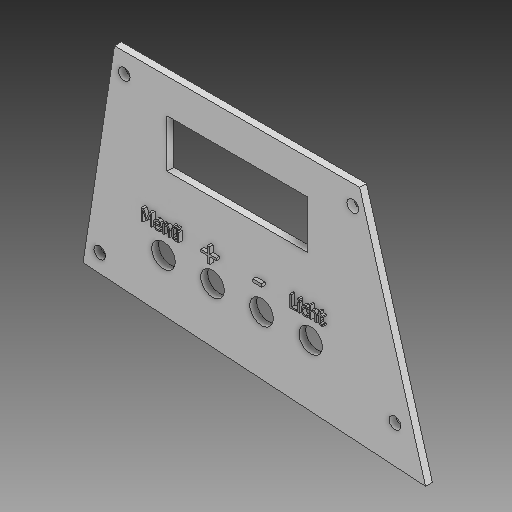
# Autodesk Inventor part: Bauteil1
Saved by Autodesk Inventor 2021 (Build 250183000, 183)
## iProperties
Created: 2021-11-26
Part Number: Bauteil1
Material: Generisch
Document SubType Name: Modeling
Designer: stroh
Density: 1 g/cm^3
Appearance: Vorgabe
Stock Number: Bedienelement
Author: stroh
Autodesk Inventor part; units mm, degrees
ref_plane "YZ Plane" through (0, 0, 0) normal (1, 0, 0) x (0, 1, 0)
ref_plane "XZ Plane" through (0, 0, 0) normal (0, 1, 0) x (-1, 0, 0)
ref_plane "XY Plane" through (0, 0, 0) normal (0, 0, 1) x (1, 0, 0)
sketch "Skizze1" plane through (0, 0, 0) normal (0, 0, 1) x (1, 0, 0)
  line L0 (-76.5913, -13.7675) -> (98.0346, -25.2043)
  line L1 (98.0346, -25.2043) -> (64.4493, 90)
  line L2 (64.4493, 90) -> (-60.5507, 90)
  line L3 (-60.5507, 90) -> (-76.5913, -13.7675)
  point P0 (0, 0)
  dimension "d0" = 175
  dimension "d1" = 120
  dimension "d2" = 105
  dimension "d3" = 125
  dimension "d5" = 70
  dimension "d12" = 90
  dimension "d14" = 90
  constraints: 8 end point
  measures "d0" distance of L0.start L0.end
  measures "d1" distance of L0.end L1.end
  measures "d2" distance of L2.end L0.start
  measures "d3" distance of L1.end L2.end
  measures "d5" angle of L1 L0
  measures "d12" vertical distance of point (0, 0) L1.end
  measures "d14" vertical distance of point (0, 0) L2.end
extrude "Extrusion1" add sketch "Skizze1" along normal blind 3.5
sketch "Skizze2" plane through (0, 0, 3.5) normal (0, 0, 1) x (1, 0, 0)
  line L0 (-33.8007, 72.5) -> (37.6993, 72.5)
  line L1 (37.6993, 72.5) -> (37.6993, 48)
  line L2 (37.6993, 48) -> (-33.8007, 48)
  line L3 (-33.8007, 48) -> (-33.8007, 72.5)
  line L4 (64.4493, 90) -> (-60.5507, 90) projected
  circle A0 centre (-35.5507, 10) radius 6.025
  circle A1 centre (-10.5507, 10) radius 6.025
  circle A2 centre (14.4493, 10) radius 6.025
  circle A3 centre (39.4493, 10) radius 6.025
  point P0 (0, 0)
  dimension "d8" = 71.5
  dimension "d9" = 24.5
  dimension "d18" = 80
  dimension "d19" = 25
  dimension "d20" = 25
  dimension "d21" = 25
  dimension "d22" = 80
  dimension "d25" = 12.05
  dimension "d26" = 12.05
  dimension "d27" = 12.05
  dimension "d28" = 12.05
  dimension "d48" = 26.75
  dimension "d49" = 26.75
  dimension "d50" = 25
  dimension "d51" = 25
  dimension "d52" = 80
  dimension "d53" = 80
  constraints: 8 end point, 4 centre point, 2 parallel, 1 horizontal, 1 perpendicular
  measures "d8" distance of L0.start L0.end
  measures "d9" distance of L2.end L0.start
  measures "d18" vertical distance of L4.end A0.centre
  measures "d19" distance of A1.centre A0.centre
  measures "d20" distance of A2.centre A1.centre
  measures "d21" distance of A2.centre A3.centre
  measures "d22" distance from line of L4 A1.centre
  measures "d25" diameter of A0
  measures "d26" diameter of A1
  measures "d27" diameter of A2
  measures "d28" diameter of A3
  measures "d48" distance from line of L4.end L3
  measures "d49" distance from line of L4.start L1
  measures "d50" horizontal distance of L4.end A0.centre
  measures "d51" horizontal distance of L4.start A3.centre
  measures "d52" distance from line of L4 A2.centre
  measures "d53" distance from line of L4 A3.centre
extrude "Extrusion2" cut sketch "Skizze2" against normal blind 5
sketch "Skizze3" plane through (0, 0, 3.5) normal (0, 0, 1) x (1, 0, 0)
  line L0 (-45.7172, 27.2505) -> (-25.2588, 27.2505) construction
  line L1 (-25.2588, 27.2505) -> (-25.2588, 20.6661) construction
  line L2 (-25.2588, 20.6661) -> (-45.7172, 20.6661) construction
  line L3 (-45.7172, 20.6661) -> (-45.7172, 27.2505) construction
  line L4 (-15.8595, 27.2834) -> (0.8474, 27.2834) construction
  line L5 (0.8474, 27.2834) -> (0.8474, 22.6055) construction
  line L6 (0.8474, 22.6055) -> (-15.8595, 22.6055) construction
  line L7 (-15.8595, 22.6055) -> (-15.8595, 27.2834) construction
  line L8 (10.9705, 24.1223) -> (26.0544, 24.1223) construction
  line L9 (26.0544, 24.1223) -> (26.0544, 18.2033) construction
  line L10 (26.0544, 18.2033) -> (10.9705, 18.2033) construction
  line L11 (10.9705, 18.2033) -> (10.9705, 24.1223) construction
  line L12 (29.9728, 27.2179) -> (48.0162, 27.2179) construction
  line L13 (48.0162, 27.2179) -> (48.0162, 20.9171) construction
  line L14 (48.0162, 20.9171) -> (29.9728, 20.9171) construction
  line L15 (29.9728, 20.9171) -> (29.9728, 27.2179) construction
  line L16 (-81.6927, 20.4062) -> (40.124, 20.4062) construction
  line L17 (-39.8693, 21.106) -> (-40.68, 21.106)
  line L18 (-40.68, 21.106) -> (-40.68, 26.3607)
  line L19 (-40.68, 26.3607) -> (-42.2718, 22.7867)
  line L20 (-42.2718, 22.7867) -> (-42.7661, 22.7867)
  line L21 (-42.7661, 22.7867) -> (-44.343, 26.3607)
  line L22 (-44.343, 26.3607) -> (-44.343, 21.106)
  line L23 (-44.343, 21.106) -> (-45.0993, 21.106)
  line L24 (-45.0993, 21.106) -> (-45.0993, 27.206)
  line L25 (-45.0993, 27.206) -> (-43.992, 27.206)
  line L26 (-43.992, 27.206) -> (-42.4695, 23.81)
  line L27 (-42.4695, 23.81) -> (-40.9964, 27.206)
  line L28 (-40.9964, 27.206) -> (-39.8693, 27.206)
  line L29 (-39.8693, 27.206) -> (-39.8693, 21.106)
  spline S0 degree 2 poles (-36.7056, 21.0022) (-37.803, 21.0022) (-39.0092, 22.2331) (-39.0092, 23.37) knots 0 0 0 1 2 2 2
  spline S1 degree 2 poles (-39.0092, 23.37) (-39.0092, 24.4872) (-37.8376, 25.812) (-36.8935, 25.812) knots 0 0 0 1 2 2 2
  spline S2 degree 2 poles (-36.8935, 25.812) (-36.4684, 25.812) (-35.8109, 25.5648) (-35.5687, 25.3028) knots 0 0 0 1 2 2 2
  spline S3 degree 2 poles (-35.5687, 25.3028) (-35.3215, 25.0408) (-35.0595, 24.2845) (-35.0595, 23.7358) knots 0 0 0 1 2 2 2
  line L30 (-35.0595, 23.7358) -> (-35.0595, 23.3156)
  line L31 (-35.0595, 23.3156) -> (-38.2282, 23.3156)
  spline S4 degree 2 poles (-38.2282, 23.3156) (-38.2282, 22.5198) (-37.4274, 21.6745) (-36.7155, 21.6745) knots 0 0 0 1 2 2 2
  spline S5 degree 2 poles (-36.7155, 21.6745) (-36.4634, 21.6745) (-35.974, 21.7882) (-35.7763, 21.8771) knots 0 0 0 1 2 2 2
  spline S6 degree 2 poles (-35.7763, 21.8771) (-35.5687, 21.976) (-35.282, 22.149) (-35.1881, 22.2281) knots 0 0 0 1 2 2 2
  line L32 (-35.1881, 22.2281) -> (-35.1436, 22.2281)
  line L33 (-35.1436, 22.2281) -> (-35.1436, 21.3878)
  spline S7 degree 2 poles (-35.1436, 21.3878) (-35.277, 21.3334) (-35.6824, 21.1752) (-35.8406, 21.1307) knots 0 0 0 1 2 2 2
  spline S8 degree 2 poles (-35.8406, 21.1307) (-36.063, 21.0664) (-36.4288, 21.0022) (-36.7056, 21.0022) knots 0 0 0 1 2 2 2
  spline S9 degree 2 poles (-35.8109, 23.9039) (-35.8208, 24.2153) (-35.9493, 24.6701) (-36.0729, 24.8233) knots 0 0 0 1 2 2 2
  spline S10 degree 2 poles (-36.0729, 24.8233) (-36.2064, 24.9963) (-36.6265, 25.1792) (-36.938, 25.1792) knots 0 0 0 1 2 2 2
  spline S11 degree 2 poles (-36.938, 25.1792) (-37.2445, 25.1792) (-37.6745, 24.9963) (-37.8525, 24.8184) knots 0 0 0 1 2 2 2
  spline S12 degree 2 poles (-37.8525, 24.8184) (-38.0255, 24.6355) (-38.2034, 24.1955) (-38.2282, 23.9039) knots 0 0 0 1 2 2 2
  line L34 (-38.2282, 23.9039) -> (-35.8109, 23.9039)
  line L35 (-30.6847, 21.106) -> (-31.4559, 21.106)
  line L36 (-31.4559, 21.106) -> (-31.4559, 23.716)
  spline S13 degree 2 poles (-31.4559, 23.716) (-31.4559, 24.0324) (-31.5152, 24.5762) (-31.6042, 24.7393) knots 0 0 0 1 2 2 2
  spline S14 degree 2 poles (-31.6042, 24.7393) (-31.6981, 24.9123) (-32.0342, 25.0804) (-32.321, 25.0804) knots 0 0 0 1 2 2 2
  spline S15 degree 2 poles (-32.321, 25.0804) (-32.6077, 25.0804) (-33.2157, 24.7739) (-33.5073, 24.5267) knots 0 0 0 1 2 2 2
  line L37 (-33.5073, 24.5267) -> (-33.5073, 21.106)
  line L38 (-33.5073, 21.106) -> (-34.2785, 21.106)
  line L39 (-34.2785, 21.106) -> (-34.2785, 25.6835)
  line L40 (-34.2785, 25.6835) -> (-33.5073, 25.6835)
  line L41 (-33.5073, 25.6835) -> (-33.5073, 25.1743)
  spline S16 degree 2 poles (-33.5073, 25.1743) (-33.1613, 25.4857) (-32.494, 25.812) (-32.1183, 25.812) knots 0 0 0 1 2 2 2
  spline S17 degree 2 poles (-32.1183, 25.812) (-31.446, 25.812) (-30.6847, 24.9222) (-30.6847, 24.0769) knots 0 0 0 1 2 2 2
  line L42 (-30.6847, 24.0769) -> (-30.6847, 21.106)
  line L43 (-26.043, 21.106) -> (-26.8141, 21.106)
  line L44 (-26.8141, 21.106) -> (-26.8141, 21.6102)
  spline S18 degree 2 poles (-26.8141, 21.6102) (-27.1701, 21.2988) (-27.8077, 20.9775) (-28.2032, 20.9775) knots 0 0 0 1 2 2 2
  spline S19 degree 2 poles (-28.2032, 20.9775) (-28.4998, 20.9775) (-29.0287, 21.1752) (-29.2215, 21.3878) knots 0 0 0 1 2 2 2
  spline S20 degree 2 poles (-29.2215, 21.3878) (-29.4193, 21.6003) (-29.6368, 22.2479) (-29.6368, 22.7125) knots 0 0 0 1 2 2 2
  line L45 (-29.6368, 22.7125) -> (-29.6368, 25.6835)
  line L46 (-29.6368, 25.6835) -> (-28.8656, 25.6835)
  line L47 (-28.8656, 25.6835) -> (-28.8656, 23.0734)
  spline S21 degree 2 poles (-28.8656, 23.0734) (-28.8656, 22.7076) (-28.8112, 22.2281) (-28.7173, 22.0501) knots 0 0 0 1 2 2 2
  spline S22 degree 2 poles (-28.7173, 22.0501) (-28.6234, 21.8722) (-28.3021, 21.7091) (-28.0005, 21.7091) knots 0 0 0 1 2 2 2
  spline S23 degree 2 poles (-28.0005, 21.7091) (-27.7188, 21.7091) (-27.0811, 22.0304) (-26.8141, 22.2627) knots 0 0 0 1 2 2 2
  line L48 (-26.8141, 22.2627) -> (-26.8141, 25.6835)
  line L49 (-26.8141, 25.6835) -> (-26.043, 25.6835)
  line L50 (-26.043, 25.6835) -> (-26.043, 21.106)
  line L51 (-26.562, 26.4497) -> (-27.3876, 26.4497)
  line L52 (-27.3876, 26.4497) -> (-27.3876, 27.2505)
  line L53 (-27.3876, 27.2505) -> (-26.562, 27.2505)
  line L54 (-26.562, 27.2505) -> (-26.562, 26.4497)
  line L55 (-28.2526, 26.4497) -> (-29.0782, 26.4497)
  line L56 (-29.0782, 26.4497) -> (-29.0782, 27.2505)
  line L57 (-29.0782, 27.2505) -> (-28.2526, 27.2505)
  line L58 (-28.2526, 27.2505) -> (-28.2526, 26.4497)
  line L59 (-6.9049, 22.8183) -> (-10.2922, 22.8183)
  line L60 (-10.2922, 22.8183) -> (-10.2922, 19.4309)
  line L61 (-10.2922, 19.4309) -> (-11.4105, 19.4309)
  line L62 (-11.4105, 19.4309) -> (-11.4105, 22.8183)
  line L63 (-11.4105, 22.8183) -> (-14.7979, 22.8183)
  line L64 (-14.7979, 22.8183) -> (-14.7979, 23.8961)
  line L65 (-14.7979, 23.8961) -> (-11.4105, 23.8961)
  line L66 (-11.4105, 23.8961) -> (-11.4105, 27.2834)
  line L67 (-11.4105, 27.2834) -> (-10.2922, 27.2834)
  line L68 (-10.2922, 27.2834) -> (-10.2922, 23.8961)
  line L69 (-10.2922, 23.8961) -> (-6.9049, 23.8961)
  line L70 (-6.9049, 23.8961) -> (-6.9049, 22.8183)
  line L71 (16.2412, 22.6636) -> (11.6999, 22.6636)
  line L72 (11.6999, 22.6636) -> (11.6999, 24.1223)
  line L73 (11.6999, 24.1223) -> (16.2412, 24.1223)
  line L74 (16.2412, 24.1223) -> (16.2412, 22.6636)
  line L75 (34.1252, 20.8461) -> (30.5907, 20.8461)
  line L76 (30.5907, 20.8461) -> (30.5907, 26.9461)
  line L77 (30.5907, 26.9461) -> (31.4014, 26.9461)
  line L78 (31.4014, 26.9461) -> (31.4014, 21.5678)
  line L79 (31.4014, 21.5678) -> (34.1252, 21.5678)
  line L80 (34.1252, 21.5678) -> (34.1252, 20.8461)
  line L81 (35.4895, 20.8461) -> (34.7183, 20.8461)
  line L82 (34.7183, 20.8461) -> (34.7183, 25.4235)
  line L83 (34.7183, 25.4235) -> (35.4895, 25.4235)
  line L84 (35.4895, 25.4235) -> (35.4895, 20.8461)
  line L85 (35.5439, 26.1848) -> (34.6689, 26.1848)
  line L86 (34.6689, 26.1848) -> (34.6689, 26.9856)
  line L87 (34.6689, 26.9856) -> (35.5439, 26.9856)
  line L88 (35.5439, 26.9856) -> (35.5439, 26.1848)
  spline S24 degree 2 poles (38.4406, 20.7423) (37.9661, 20.7423) (37.1801, 21.0339) (36.8983, 21.3305) knots 0 0 0 1 2 2 2
  spline S25 degree 2 poles (36.8983, 21.3305) (36.6166, 21.6222) (36.3051, 22.5218) (36.3051, 23.1249) knots 0 0 0 1 2 2 2
  spline S26 degree 2 poles (36.3051, 23.1249) (36.3051, 23.728) (36.6264, 24.6079) (36.8983, 24.9045) knots 0 0 0 1 2 2 2
  spline S27 degree 2 poles (36.8983, 24.9045) (37.1702, 25.206) (37.976, 25.5273) (38.4406, 25.5273) knots 0 0 0 1 2 2 2
  spline S28 degree 2 poles (38.4406, 25.5273) (38.8163, 25.5273) (39.5183, 25.3148) (39.7901, 25.1764) knots 0 0 0 1 2 2 2
  line L89 (39.7901, 25.1764) -> (39.7901, 24.3113)
  line L90 (39.7901, 24.3113) -> (39.7457, 24.3113)
  spline S29 degree 2 poles (39.7457, 24.3113) (39.6616, 24.3805) (39.4046, 24.5585) (39.2217, 24.6524) knots 0 0 0 1 2 2 2
  spline S30 degree 2 poles (39.2217, 24.6524) (39.0585, 24.7315) (38.6235, 24.8551) (38.4258, 24.8551) knots 0 0 0 1 2 2 2
  spline S31 degree 2 poles (38.4258, 24.8551) (37.8277, 24.8551) (37.101, 23.9504) (37.101, 23.1249) knots 0 0 0 1 2 2 2
  spline S32 degree 2 poles (37.101, 23.1249) (37.101, 22.3192) (37.8029, 21.4145) (38.4258, 21.4145) knots 0 0 0 1 2 2 2
  spline S33 degree 2 poles (38.4258, 21.4145) (38.8015, 21.4145) (39.4837, 21.726) (39.7457, 21.9682) knots 0 0 0 1 2 2 2
  line L91 (39.7457, 21.9682) -> (39.7901, 21.9682)
  line L92 (39.7901, 21.9682) -> (39.7901, 21.1031)
  spline S34 degree 2 poles (39.7901, 21.1031) (39.6764, 21.0487) (39.3304, 20.8955) (39.192, 20.8609) knots 0 0 0 1 2 2 2
  spline S35 degree 2 poles (39.192, 20.8609) (38.9943, 20.8016) (38.6828, 20.7423) (38.4406, 20.7423) knots 0 0 0 1 2 2 2
  line L93 (44.0858, 20.8461) -> (43.3147, 20.8461)
  line L94 (43.3147, 20.8461) -> (43.3147, 23.4561)
  spline S36 degree 2 poles (43.3147, 23.4561) (43.3147, 23.7725) (43.2554, 24.3162) (43.1664, 24.4794) knots 0 0 0 1 2 2 2
  spline S37 degree 2 poles (43.1664, 24.4794) (43.0725, 24.6524) (42.7363, 24.8205) (42.4496, 24.8205) knots 0 0 0 1 2 2 2
  spline S38 degree 2 poles (42.4496, 24.8205) (42.1629, 24.8205) (41.5549, 24.514) (41.2632, 24.2668) knots 0 0 0 1 2 2 2
  line L95 (41.2632, 24.2668) -> (41.2632, 20.8461)
  line L96 (41.2632, 20.8461) -> (40.4921, 20.8461)
  line L97 (40.4921, 20.8461) -> (40.4921, 27.2179)
  line L98 (40.4921, 27.2179) -> (41.2632, 27.2179)
  line L99 (41.2632, 27.2179) -> (41.2632, 24.9144)
  spline S39 degree 2 poles (41.2632, 24.9144) (41.6093, 25.2258) (42.2766, 25.5521) (42.6523, 25.5521) knots 0 0 0 1 2 2 2
  spline S40 degree 2 poles (42.6523, 25.5521) (43.3246, 25.5521) (44.0858, 24.6623) (44.0858, 23.817) knots 0 0 0 1 2 2 2
  line L100 (44.0858, 23.817) -> (44.0858, 20.8461)
  spline S41 degree 2 poles (46.5525, 20.7571) (45.9247, 20.7571) (45.2179, 21.4739) (45.2179, 22.25) knots 0 0 0 1 2 2 2
  line L101 (45.2179, 22.25) -> (45.2179, 24.7859)
  line L102 (45.2179, 24.7859) -> (44.6988, 24.7859)
  line L103 (44.6988, 24.7859) -> (44.6988, 25.4235)
  line L104 (44.6988, 25.4235) -> (45.2179, 25.4235)
  line L105 (45.2179, 25.4235) -> (45.2179, 26.7384)
  line L106 (45.2179, 26.7384) -> (45.989, 26.7384)
  line L107 (45.989, 26.7384) -> (45.989, 25.4235)
  line L108 (45.989, 25.4235) -> (47.4077, 25.4235)
  line L109 (47.4077, 25.4235) -> (47.4077, 24.7859)
  line L110 (47.4077, 24.7859) -> (45.989, 24.7859)
  line L111 (45.989, 24.7859) -> (45.989, 22.6059)
  spline S42 degree 2 poles (45.989, 22.6059) (45.989, 22.2598) (46.0137, 21.8792) (46.0978, 21.7161) knots 0 0 0 1 2 2 2
  spline S43 degree 2 poles (46.0978, 21.7161) (46.167, 21.5727) (46.4784, 21.4294) (46.7453, 21.4294) knots 0 0 0 1 2 2 2
  spline S44 degree 2 poles (46.7453, 21.4294) (46.9332, 21.4294) (47.2841, 21.5431) (47.3632, 21.5777) knots 0 0 0 1 2 2 2
  line L112 (47.3632, 21.5777) -> (47.4077, 21.5777)
  line L113 (47.4077, 21.5777) -> (47.4077, 20.8856)
  spline S45 degree 2 poles (47.4077, 20.8856) (47.1902, 20.8263) (46.7453, 20.7571) (46.5525, 20.7571) knots 0 0 0 1 2 2 2
  point P0 (0, 0)
  constraints: 2 end point, 1 parallel, 8 other
extrude "Extrusion3" add sketch "Skizze3" along normal blind 1.75
sketch "Skizze4" plane through (0, 0, 3.5) normal (0, 0, 1) x (1, 0, 0)
  circle A0 centre (-55.5507, 80) radius 3
  circle A1 centre (60.9493, 80) radius 3
  circle A2 centre (-68.0507, -5) radius 3
  circle A3 centre (82.4493, -5) radius 3
  line L0 (64.4493, 90) -> (-60.5507, 90) projected
  point P0 (0, 0)
  dimension "d33" = 6
  dimension "d34" = 6
  dimension "d35" = 6
  dimension "d36" = 6
  dimension "d37" = 10
  dimension "d38" = 10
  dimension "d39" = 5
  dimension "d40" = 3.5
  dimension "d41" = 95
  dimension "d43" = 95
  dimension "d44" = 7.5
  dimension "d45" = 18
  constraints: 4 centre point
  measures "d33" diameter of A2
  measures "d34" diameter of A3
  measures "d35" diameter of A0
  measures "d36" diameter of A1
  measures "d37" distance from line of L0 A0.centre
  measures "d38" distance from line of L0 A1.centre
  measures "d39" horizontal distance of L0.end A0.centre
  measures "d40" horizontal distance of L0.start A1.centre
  measures "d41" vertical distance of L0.end A2.centre
  measures "d43" vertical distance of L0.start A3.centre
  measures "d44" horizontal distance of L0.end A2.centre
  measures "d45" horizontal distance of L0.start A3.centre
extrude "Extrusion4" cut sketch "Skizze4" against normal blind 5
